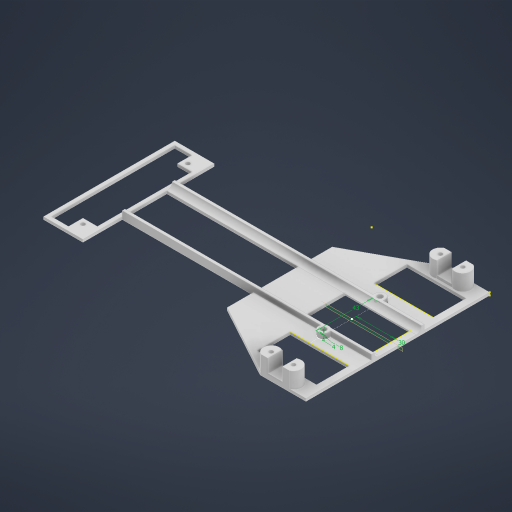
# Autodesk Inventor part: Part4
Saved by Autodesk Inventor 2023 (Build 270158000, 158)
## iProperties
Created: 2023-02-02
Part Number: Part4
Material: Generic
Document SubType Name: Modeling
Designer: aniela
Density: 1 g/cm^3
Appearance: Default
Author: aniela
Autodesk Inventor part; units mm, degrees
ref_plane "YZ Plane" through (0, 0, 0) normal (1, 0, 0) x (0, 1, 0)
ref_plane "XZ Plane" through (0, 0, 0) normal (0, 1, 0) x (-1, 0, 0)
ref_plane "XY Plane" through (0, 0, 0) normal (0, 0, 1) x (1, 0, 0)
sketch "Sketch1" plane through (0, 0, 0) normal (0, 1, 0) x (-1, 0, 0)
  line L0 (0, 0) -> (35, 0) construction
  line L1 (90, 30) -> (90, 110) construction
  line L2 (35, 140) -> (0, 140)
  line L3 (0, 140) -> (0, 0)
  line L4 (0, 0) -> (35, 0) construction
  line L5 (35, 0) -> (35, 140) construction
  line L6 (35, 140) -> (0, 140) construction
  line L7 (0, 140) -> (0, 0) construction
  line L8 (90, 110) -> (35, 140) construction
  line L9 (35, 0) -> (90, 30) construction
  line L10 (35, 140) -> (90, 110) construction
  line L11 (35, 0) -> (90, 30) construction
  line L12 (90, 110) -> (90, 30) construction
  line L13 (35, 0) -> (90, 30)
  line L14 (90, 30) -> (90, 110)
  line L15 (90, 110) -> (35, 140)
  line L16 (5, 127) -> (50, 127) construction
  line L17 (50, 127) -> (50, 102) construction
  line L18 (50, 102) -> (5, 102) construction
  line L19 (5, 102) -> (5, 127) construction
  line L20 (50, 127) -> (50, 102) construction
  line L21 (50, 102) -> (5, 102) construction
  line L22 (50, 127) -> (50, 102)
  line L23 (50, 127) -> (5, 127)
  line L24 (50, 102) -> (5, 102)
  line L25 (5, 102) -> (5, 127)
  line L26 (35, 0) -> (0, 0) construction
  line L27 (5, 13) -> (50, 13) construction
  line L28 (50, 13) -> (50, 38) construction
  line L29 (50, 38) -> (5, 38) construction
  line L30 (5, 38) -> (5, 13) construction
  line L31 (50, 38) -> (5, 38) construction
  line L32 (5, 38) -> (5, 13) construction
  line L33 (5, 13) -> (50, 13) construction
  line L34 (50, 13) -> (50, 38) construction
  line L35 (5, 13) -> (50, 13) construction
  line L36 (50, 13) -> (50, 38) construction
  line L37 (50, 38) -> (5, 38) construction
  line L38 (5, 38) -> (5, 13) construction
  line L39 (50, 38) -> (50, 13)
  line L40 (50, 13) -> (5, 13)
  line L41 (5, 13) -> (5, 38)
  line L42 (5, 38) -> (50, 38)
  line L43 (9.9818, 0) -> (0, 0) construction
  line L44 (0, 0) -> (0, 55) construction
  line L45 (0, 55) -> (9.9818, 55) construction
  line L46 (9.9818, 55) -> (9.9818, 0) construction
  line L47 (5, 55) -> (55, 55) construction
  line L48 (55, 55) -> (55, 92) construction
  line L49 (5, 92) -> (5, 55) construction
  line L50 (5, 92) -> (5, 55) construction
  line L51 (5, 55) -> (55, 55) construction
  line L52 (55, 55) -> (55, 92) construction
  line L53 (55, 92) -> (55, 55) construction
  line L54 (55, 55) -> (5, 55)
  line L55 (35, 0) -> (0, 0)
  line L56 (55, 55) -> (55, 85)
  line L57 (55, 85) -> (5, 85)
  line L58 (5, 55) -> (5, 85)
  line L59 (90, 30) -> (90, 0) construction
  line L60 (90, 110) -> (90, 140) construction
  dimension "d144" = 13
  dimension "d145" = 25
  dimension "d146" = 17
  dimension "d147" = 30
  dimension "d148" = 17
  dimension "d149" = 25
  dimension "d150" = 13
  dimension "d151" = 5
  dimension "d152" = 45
  dimension "d153" = 50
  dimension "d157" = 80
  dimension "d158" = 35
  dimension "d159" = 90
  constraints: 122 end point, 23 collinear, 16 parallel, 9 perpendicular, 9 point on line, 8 horizontal, 2 equal length, 1 vertical
  measures "d144" distance between parallel lines of L0 L27
  measures "d145" distance between parallel lines of L27 L29
  measures "d146" distance between parallel lines of L29 L47
  measures "d147" distance of L47.start L57.end
  measures "d148" distance between parallel lines of L57 L18
  measures "d149" distance between parallel lines of L18 L16
  measures "d150" distance between parallel lines of L16 L2
  measures "d151" distance between parallel lines of L32 L3
  measures "d152" distance between parallel lines of L30 L28
  measures "d153" distance between parallel lines of L58 L52
  measures "d157" distance of L1.start L1.end
  measures "d158" distance of L0.start L4.end
  measures "d159" distance between parallel lines of L3 L12
sketch "Sketch2" plane through (0, 0, 0) normal (0, 1, 0) x (-1, 0, 0)
  point P0 (0, 0)
sketch "Sketch3" plane through (0, 0, 0) normal (0, 1, 0) x (-1, 0, 0)
  point P0 (0, 0)
sketch "Sketch4" plane through (0, 0, 0) normal (0, 1, 0) x (-1, 0, 0)
  line L0 (0, 0) -> (35.5492, 0)
  line L1 (0, 0) -> (35, 0) construction
  line L2 (35, 0) -> (90, 30) construction
  line L3 (35, 0) -> (0, 0)
  constraints: 4 end point, 2 horizontal
extrude "Extrusion1" add sketch "Sketch1" along normal blind 2
sketch "Sketch5" plane through (0, 2, 0) normal (0, 1, 0) x (1, 0, 0)
  line L0 (0, 0) -> (-35, 0) projected
  line L1 (-15, 0) -> (-32, 0)
  line L2 (-32, 0) -> (-32, -11)
  line L3 (-32, -11) -> (-15, -11)
  line L4 (-15, -11) -> (-15, 0)
  line L5 (-32, 0) -> (-15, 0)
  line L6 (-15, 0) -> (-15, -11)
  line L7 (-15, -11) -> (-32, -11)
  line L8 (-32, -11) -> (-32, 0)
  line L9 (-35, -140) -> (0, -140) projected
  line L10 (-15, -140) -> (-32, -140)
  line L11 (-32, -140) -> (-32, -129)
  line L12 (-32, -129) -> (-15, -129)
  line L13 (-15, -129) -> (-15, -140)
  line L14 (-32, -129) -> (-15, -129)
  line L15 (-15, -129) -> (-15, -140)
  line L16 (-15, -140) -> (-32, -140)
  line L17 (-32, -140) -> (-32, -129)
  dimension "d22" = 17
  dimension "d23" = 11
  dimension "d24" = 11
  constraints: 32 end point, 8 parallel, 4 horizontal, 4 perpendicular, 4 point on line
  measures "d22" distance of L3.end L2.end
  measures "d23" distance of L2.end L1.end
  measures "d24" distance of L10.end L11.end
extrude "Extrusion2" add sketch "Sketch5" along normal blind 2
sketch "Sketch6" plane through (0, 4, 0) normal (0, 1, 0) x (1, 0, 0)
  line L0 (-32, 0) -> (-32, -11) projected
  line L1 (-32, 0) -> (-29, 0)
  line L2 (-29, 0) -> (-29, -11)
  line L3 (-29, -11) -> (-32, -11)
  line L4 (-32, -11) -> (-32, 0)
  line L5 (-15, -11) -> (-15, 0) projected
  line L6 (-32, -11) -> (-15, -11) projected
  line L7 (-15, 0) -> (-18, 0)
  line L8 (-18, 0) -> (-18, -11)
  line L9 (-18, -11) -> (-15, -11)
  line L10 (-15, -11) -> (-15, 0)
  line L11 (-32, -11) -> (-32, 0)
  line L12 (0, 0) -> (-35, 0) projected
  line L13 (-32, -11) -> (-15, -11)
  line L14 (-32, 0) -> (-15, 0)
  line L15 (-15, -129) -> (-15, -140) projected
  line L16 (-32, -129) -> (-15, -129) projected
  line L17 (-15, -140) -> (-18, -140)
  line L18 (-18, -140) -> (-18, -129)
  line L19 (-18, -129) -> (-15, -129)
  line L20 (-15, -129) -> (-15, -140)
  line L21 (-32, -129) -> (-29, -129)
  line L22 (-29, -129) -> (-29, -140)
  line L23 (-29, -140) -> (-32, -140)
  line L24 (-32, -140) -> (-32, -129)
  line L25 (-35, -140) -> (-32, -140) projected
  line L26 (-32, -140) -> (-32, -129)
  line L27 (-32, -129) -> (-15, -129)
  line L28 (-18, -129) -> (-18, -140)
  line L29 (-35, -140) -> (0, -140) projected
  line L30 (-29, -129) -> (-29, -140)
  dimension "d27" = 3
  dimension "d28" = 3
  constraints: 46 end point, 11 equal length, 8 perpendicular, 4 horizontal, 4 point on line
  measures "d27" distance of L2.end L3.end
  measures "d28" distance of L9.end L8.end
extrude "Extrusion3" add sketch "Sketch6" along normal blind 10 contours L15 L17 L18 L16 | L22 L23 L24 L16
sketch "Sketch7" plane through (0, 4, 0) normal (0, 1, 0) x (1, 0, 0)
  line L0 (-15, -11) -> (-15, 0) projected
  line L1 (-32, -11) -> (-15, -11) projected
  line L2 (-15, 0) -> (-18, 0)
  line L3 (-18, 0) -> (-18, -11)
  line L4 (-18, -11) -> (-15, -11)
  line L5 (-15, -11) -> (-15, 0)
  line L6 (-18, -11) -> (-15, -11)
  line L7 (-15, -11) -> (-15, 0)
  line L8 (-15, 0) -> (-18, 0)
  line L9 (-18, 0) -> (-18, -11)
  line L10 (-32, 0) -> (-32, -11) projected
  line L11 (-32, 0) -> (-29, 0)
  line L12 (-29, 0) -> (-29, -11)
  line L13 (-29, -11) -> (-32, -11)
  line L14 (-32, -11) -> (-32, 0)
  line L15 (-18, -11) -> (-29, -11)
  point P0 (0, 0)
  dimension "d31" = 3
  dimension "d32" = 3
  constraints: 26 end point, 6 parallel, 4 perpendicular, 3 horizontal, 2 point on line
  measures "d31" distance of L4.end L3.end
  measures "d32" distance of L12.end L13.end
extrude "Extrusion4" add sketch "Sketch7" along normal blind 10
sketch "Sketch8" plane through (0, 2, 0) normal (0, 1, 0) x (1, 0, 0)
  line L0 (-80, -55) -> (-70, -55)
  line L1 (-70, -55) -> (-70, -85)
  line L2 (-70, -85) -> (-80, -85)
  line L3 (-80, -85) -> (-80, -55)
  circle A0 centre (-75, -60) radius 1.5
  circle A1 centre (-75, -80) radius 1.5
  point P0 (0, 0)
  dimension "d35" = 10
  dimension "d36" = 30
  dimension "d37" = 3
  dimension "d38" = 3
  constraints: 8 end point, 2 centre point, 2 parallel, 1 horizontal, 1 perpendicular
  measures "d35" distance of L1.end L2.end
  measures "d36" distance of L0.end L1.end
  measures "d37" diameter of A0
  measures "d38" diameter of A1
extrude "Extrusion5" cut sketch "Sketch8" along normal blind 2
sketch "Sketch11" plane through (0, 14, 0) normal (0, 1, 0) x (1, 0, 0)
  line L0 (-15, 0) -> (-15, -11) projected
  circle A0 centre (-15, -5.5) radius 3
  line L1 (-32, -11) -> (-32, 0) projected
  circle A1 centre (-32, -5.5) radius 3
  point P0 (0, 0)
  point P1 (-15, -2.5)
  point P2 (-15, -8.5)
  point P3 (-32, -2.5)
  point P4 (-32, -8.5)
  dimension "d55" = 6
  dimension "d56" = 6
  constraints: 2 centre point, 2 midpoint
  measures "d55" diameter of A0
  measures "d56" diameter of A1
extrude "Extrusion6" add sketch "Sketch11" against normal blind 12 contours A0 L0 | A1 L1 picked at (-13.8765, -5.0912) picked at (-33.7524, -6.0681)
sketch "Sketch12" plane through (0, 14, 0) normal (0, 1, 0) x (1, 0, 0)
  arc A0 (-15, -8.5) -> (-15, -2.5) centre (-15, -5.5) ccw projected
  circle A1 centre (-15, -5.5) radius 2
  point P0 (0, 0)
  dimension "d59" = 4
  constraints: 1 centre point, 1 coincident
  measures "d59" diameter of A1
sketch "Sketch13" plane through (0, 14, 0) normal (0, 1, 0) x (1, 0, 0)
  arc A0 (-32, -2.5) -> (-32, -8.5) centre (-32, -5.5) ccw projected
  circle A1 centre (-32, -5.5) radius 2
  point P0 (0, 0)
  dimension "d60" = 4
  constraints: 1 centre point, 1 coincident
  measures "d60" diameter of A1
hole "Hole3" at (-32, 14, 5.5) direction (0, -1, 0) diameter 3 end through all
hole "Hole4" at (-15, 14, 5.5) direction (0, -1, 0) diameter 3 end through all
sketch "Sketch14" plane through (0, 0, 0) normal (0, -1, 0) x (1, 0, 0)
  circle A0 centre (-15, 5.5) radius 1.5 projected
  circle A1 centre (-15, 5.5) radius 2
  circle A2 centre (-32, 5.5) radius 1.5 projected
  circle A3 centre (-32, 5.5) radius 2
  circle A4 centre (-15, 5.5) radius 2
  point P0 (0, 0)
  constraints: 3 centre point, 3 coincident, 1 concentric
extrude "Extrusion7" add sketch "Sketch14" against normal blind 3 contours A0 | A2
sketch "Sketch15" plane through (0, 14, 0) normal (0, 1, 0) x (1, 0, 0)
  line L0 (-15, -140) -> (-15, -129) projected
  arc A0 (-12.6021, -140) -> (-17.3979, -140) centre (-15, -134.5) ccw
  line L1 (-18, -129) -> (-18, -140) projected
  line L2 (-15, -140) -> (0, -140) projected
  line L3 (-18, -140) -> (-15, -140) projected
  arc A1 (-29, -129.3038) -> (-34.3979, -140) centre (-32, -134.5) ccw
  line L4 (-32, -129) -> (-32, -140) projected
  line L5 (-29, -140) -> (-18, -140) projected
  line L6 (-32, -140) -> (-29, -140) projected
  line L7 (-35, -140) -> (-32, -140) projected
  line L8 (-90, -110) -> (-35, -140) projected
  line L9 (-29, -140) -> (-29, -129) projected
  point P0 (0, 0)
  point P1 (-29.6021, -140)
  point P2 (-18, -129.3038)
  point P3 (-18, -139.6962)
  dimension "d138" = 12
  dimension "d139" = 12
  constraints: 5 point on line, 4 point on circle, 3 midpoint, 2 centre point, 1 horizontal alignment
  measures "d138" diameter of A0
  measures "d139" diameter of A1
extrude "Extrusion8" add sketch "Sketch15" against normal blind 12 contours L2 L3 A0 L1 | L9 L6 L7 A1
sketch "Sketch19" plane through (0, 0, 0) normal (0, -1, 0) x (1, 0, 0)
  point P0 (0, 0)
sketch "Sketch20" plane through (0, 14, 0) normal (0, 1, 0) x (1, 0, 0)
  circle A0 centre (-32, -134.5) radius 2 projected
  circle A1 centre (-32, -134.5) radius 2
  circle A2 centre (-15, -134.5) radius 2 projected
  circle A3 centre (-15, -134.5) radius 2
  point P0 (0, 0)
  constraints: 2 centre point, 2 coincident
extrude "Extrusion10" add sketch "Sketch20" against normal up to surface (14 mm away)
sketch "Sketch21" plane through (0, 0, 0) normal (0, -1, 0) x (1, 0, 0)
  point P0 (0, 0)
sketch "Sketch22" plane through (0, 14, 0) normal (0, 1, 0) x (1, 0, 0)
  arc A0 (-12.6021, -140) -> (-17.3979, -129) centre (-15, -134.5) ccw projected
  circle A1 centre (-15, -134.5) radius 1.5
  arc A2 (-32, -131.4998) -> (-32, -137.5002) centre (-32, -134.5) ccw projected
  circle A3 centre (-32, -134.5) radius 1.5
  point P0 (0, 0)
  point P1 (-15, -137.5)
  point P2 (-15, -131.5)
  dimension "d100" = 3
  dimension "d101" = 3
  constraints: 2 centre point, 2 coincident
  measures "d100" diameter of A1
  measures "d101" diameter of A3
extrude "Extrusion11" cut sketch "Sketch22" against normal blind 12
sketch "Sketch23" plane through (0, 14, 0) normal (0, 1, 0) x (1, 0, 0)
  arc A0 (-32, -131.4998) -> (-32, -137.5002) centre (-32, -134.5) ccw projected
  circle A1 centre (-32, -134.5) radius 1.5
  point P0 (0, 0)
  dimension "d104" = 3
  constraints: 1 centre point, 1 coincident
  measures "d104" diameter of A1
extrude "Extrusion12" cut sketch "Sketch23" against normal blind 12
sketch "Sketch24" plane through (0, 2, 0) normal (0, 1, 0) x (1, 0, 0)
  point P0 (0, 0)
sketch "Sketch25" plane through (0, 2, 0) normal (0, 1, 0) x (1, 0, 0)
  line L0 (-90, -110) -> (-35, -140) projected
  line L1 (-90, -30) -> (-90, -110) projected
  line L2 (-90, -90) -> (-90, -50)
  line L3 (-90, -50) -> (-190, -50)
  line L4 (-190, -50) -> (-190, -90)
  line L5 (-190, -90) -> (-91.3182, -90)
  line L6 (-91.3182, -90) -> (-90, -90)
  line L7 (-90, -84) -> (-190, -84)
  line L8 (-90, -56) -> (-190, -56)
  point P0 (0, 0)
  dimension "d117" = 40
  dimension "d118" = 100
  constraints: 14 end point, 6 perpendicular, 6 point on line
  measures "d117" distance of L2.start L2.end
  measures "d118" distance of L2.end L3.end
extrude "Extrusion13" add sketch "Sketch25" against normal blind 2 contours L1 L8 L4 L3 | L1 L6 L5 L4 L7
sketch "Sketch26" plane through (0, 2, 0) normal (0, 1, 0) x (1, 0, 0)
  line L0 (-190, -90) -> (-190, -84) projected
  line L1 (-190, -90) -> (-90, -90)
  line L2 (-90, -90) -> (-90, -88)
  line L3 (-90, -88) -> (-190, -88)
  line L4 (-190, -88) -> (-190, -90)
  line L5 (-90, -30) -> (-90, -50) projected
  line L6 (-190, -56) -> (-190, -50) projected
  line L7 (-90, -50) -> (-190, -50)
  line L8 (-190, -50) -> (-190, -52)
  line L9 (-190, -52) -> (-90, -52)
  line L10 (-90, -52) -> (-90, -50)
  point P0 (0, 0)
  dimension "d121" = 2
  dimension "d122" = 2
  constraints: 16 end point, 4 parallel, 2 horizontal, 2 perpendicular, 1 point on line
  measures "d121" distance of L2.end L1.end
  measures "d122" distance of L8.end L7.end
extrude "Extrusion14" add sketch "Sketch26" along normal blind 4
fillet "Fillet5" radius 4 1 edges at (-140, 2, 52)
fillet "Fillet6" radius 4 1 edges at (-140, 2, 88)
sketch "Sketch27" plane through (0, 2, 0) normal (0, 1, 0) x (1, 0, 0)
  line L0 (-190, -50) -> (-90, -50) projected
  line L1 (-90, -90) -> (-190, -90) projected
  line L2 (-220, -120) -> (-190, -120)
  line L3 (-190, -120) -> (-190, -20)
  line L4 (-190, -20) -> (-220, -20)
  line L5 (-220, -20) -> (-220, -120)
  line L6 (-190, -117) -> (-220, -117)
  line L7 (-220, -117) -> (-220, -120)
  line L8 (-220, -120) -> (-190, -120)
  line L9 (-190, -120) -> (-190, -117)
  line L10 (-220, -117) -> (-217, -117)
  line L11 (-217, -117) -> (-217, -20)
  line L12 (-217, -20) -> (-220, -20)
  line L13 (-220, -20) -> (-220, -117)
  line L14 (-190, -20) -> (-220, -20)
  line L15 (-220, -20) -> (-220, -23)
  line L16 (-220, -23) -> (-190, -23)
  line L17 (-190, -23) -> (-190, -20)
  line L18 (-190, -20) -> (-193, -20)
  line L19 (-193, -20) -> (-193, -120)
  line L20 (-193, -120) -> (-190, -120)
  line L21 (-190, -120) -> (-190, -20)
  line L22 (-190, -106) -> (-204, -106)
  line L23 (-204, -106) -> (-204, -120)
  line L24 (-204, -120) -> (-190, -120)
  line L25 (-190, -120) -> (-190, -106)
  line L26 (-190, -20) -> (-204, -20)
  line L27 (-204, -20) -> (-204, -34)
  line L28 (-204, -34) -> (-190, -34)
  line L29 (-190, -34) -> (-190, -20)
  point P0 (0, 0)
  point P1 (-217, -23)
  point P2 (-204, -23)
  point P3 (-193, -34)
  point P4 (-193, -106)
  point P5 (-204, -117)
  dimension "d127" = 3
  dimension "d128" = 3
  dimension "d129" = 3
  dimension "d130" = 14
  dimension "d131" = 14
  constraints: 56 end point, 14 parallel, 7 horizontal, 7 perpendicular, 7 point on line, 1 coincident
  measures "d127" distance of L12.end L11.end
  measures "d128" distance of L15.end L14.end
  measures "d129" distance of L20.end L19.end
  measures "d130" distance of L24.end L23.end
  measures "d131" distance of L27.end L26.end
extrude "Extrusion15" add sketch "Sketch27" against normal blind 2 contours L5 L6 L23 L2 | L23 L6 L19 L2 | L5 L16 L11 L6 | L19 L6 L3 L2 | L23 L22 L19 L6 | L5 L4 L11 L16 | L19 L22 L3 L6 | L11 L4 L27 L16 | L19 L28 L3 L22 | L27 L4 L19 L16 | L16 L19 L28 L27 | L19 L16 L3 L28 | L19 L4 L3 L16
sketch "Sketch28" plane through (0, 2, 0) normal (0, 1, 0) x (1, 0, 0)
  line L0 (-190, -20) -> (-190, -50) projected
  circle A0 centre (-200, -30) radius 0.75
  line L1 (-190, -90) -> (-190, -120) projected
  circle A1 centre (-200, -110) radius 0.75
  point P0 (0, 0)
  point P1 (-190, -30)
  point P2 (-190, -110)
  dimension "d134" = 1.5
  dimension "d135" = 1.5
  constraints: 3 coincident, 2 centre point, 2 point on line
  measures "d134" diameter of A0
  measures "d135" diameter of A1
extrude "Extrusion16" cut sketch "Sketch28" against normal blind 2
ref_plane "Work Plane1" through (-55, 2, 70) normal (0, 0, -1) x (1, 0, 0)
mirror "Mirror1" about plane through (-55, 2, 70) normal (0, 0, -1) of "Extrusion8", "Extrusion11"
sketch "Sketch29" plane through (0, 2, 0) normal (0, 1, 0) x (1, 0, 0)
  circle A0 centre (-200, -30) radius 0.75 projected
  circle A1 centre (-200, -30) radius 1.5
  circle A2 centre (-200, -109.9594) radius 1.5
  point P0 (0, 0)
  dimension "d140" = 3
  dimension "d141" = 3
  constraints: 2 centre point, 1 coincident
  measures "d140" diameter of A1
  measures "d141" diameter of A2
extrude "Extrusion17" cut sketch "Sketch29" against normal blind 10 contours A0 | A1 | A2
sketch "Sketch30" plane through (0, 2, 0) normal (0, 1, 0) x (1, 0, 0)
  point P0 (0, 0)
sketch "Sketch31" plane through (0, 2, 0) normal (0, 1, 0) x (1, 0, 0)
  line L0 (-35, -91.5) -> (-35, -48.5) construction
  line L1 (-5, -55) -> (-5, -85) projected
  line L2 (-35, -91.5) -> (-35, -102) construction
  line L3 (-50, -102) -> (-5, -102) projected
  line L4 (-35, -48.5) -> (-35, -38) construction
  line L5 (-5, -38) -> (-50, -38) projected
  circle A0 centre (-35, -91.5) radius 2
  circle A1 centre (-35, -48.5) radius 2
  circle A2 centre (-35, -91.5) radius 4
  circle A3 centre (-35, -48.5) radius 4
  point P0 (0, 0)
  point P1 (-35, -70)
  dimension "d160" = 43
  dimension "d161" = 30
  dimension "d162" = 4
  dimension "d163" = 8
  constraints: 6 coincident, 6 end point, 4 centre point, 3 point on line, 2 vertical, 1 collinear, 1 midpoint
  measures "d160" distance of L0.start L0.end
  measures "d161" distance from line of L1 point (-35, -70)
  measures "d162" diameter of A0
  measures "d163" diameter of A2
extrude "Extrusion18" add sketch "Sketch31" along normal blind 4 contours A0 | A1 | A2 | A3
hole "Hole7" at (-35, 2, 91.5) at (-35, 2, 48.5) direction (0, 1, 0) diameter 4 depth 19.05 tip angle 118
hole "Hole8" at (-35, 2, 91.5) at (-35, 2, 48.5) direction (0, -1, 0) diameter 4 depth 19.05 tip angle 118
sketch "Sketch32" plane through (-90, 2, 90) normal (1, 0, 0) x (0, 0, -1)
  line L0 (0, 4) -> (0, 0)
  line L1 (-50, 0) -> (90, 0) projected
  line L2 (0, 4) -> (2, 4) projected
  line L3 (0, 4) -> (2, 4)
  arc A0 (2, 4) -> (5.993, 0) centre (5.993, 3.993) ccw
  line L4 (0, 0) -> (0, 4) projected
  line L5 (0, 0) -> (5.993, 0)
  point P0 (90, -2)
  constraints: 6 end point, 2 collinear, 2 point on circle, 2 point on line, 2 tangent, 1 centre point, 1 vertical
extrude "Extrusion19" add sketch "Sketch32" along normal blind 90
sketch "Sketch33" plane through (-90, 2, 50) normal (1, 0, 0) x (0, 0, -1)
  point P0 (50, -2)
sketch "Sketch34" plane through (-90, 2, 50) normal (1, 0, 0) x (0, 0, -1)
  point P0 (50, -2)
sketch "Sketch35" plane through (-90, 2, 50) normal (1, 0, 0) x (0, 0, -1)
  point P0 (50, -2)
sketch "Sketch36" plane through (-90, 2, 50) normal (1, 0, 0) x (0, 0, -1)
  line L0 (-2, 4) -> (0, 4) projected
  line L1 (-2, 4) -> (0, 4)
  line L2 (0, 0) -> (0, 4) projected
  line L3 (0, 4) -> (0, 0)
  arc A0 (-6, 0) -> (-2, 4) centre (-6, 4) ccw projected
  arc A1 (-6, 0) -> (-2, 4) centre (-6, 4) ccw
  line L4 (0, 0) -> (-6, 0)
  line L5 (-2.5, 0) -> (5.5, 0) projected
  line L6 (0, 0) -> (-6, 0) projected
  line L7 (-6, 0) -> (0, 0)
  point P0 (50, -2)
  constraints: 8 end point, 3 point on circle, 2 perpendicular, 2 tangent, 1 centre point, 1 collinear, 1 horizontal
extrude "Extrusion20" add sketch "Sketch36" along normal blind 90
hole "Hole9" at (-35, 2, 91.5) direction (0, 1, 0) diameter 4 depth 19.05 tip angle 118
hole "Hole10" at (-35, 2, 48.5) direction (0, 1, 0) diameter 4 depth 19.05 tip angle 118
body "Solid1"
